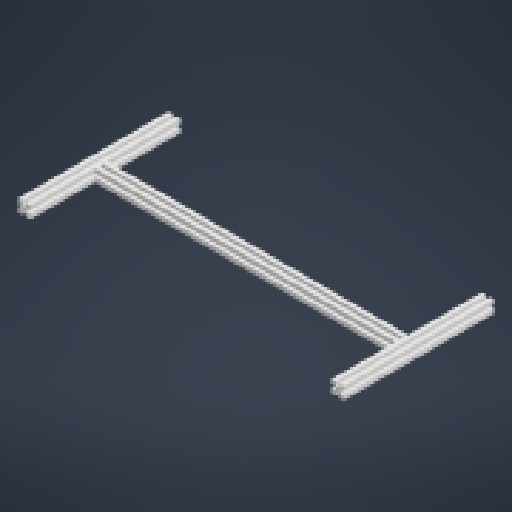
# Autodesk Inventor part: grabber
Saved by Autodesk Inventor 2024 (Build 280153000, 153)
## iProperties
Created: 2023-09-19
Part Number: grabber
Material: 일반
Document SubType Name: Modeling
Designer: 6gioc
Mass: 449.19 g
Surface Area: 2006.93 cm^2
Volume: 449.19 cm^3
Density: 1 g/cm^3
Appearance: 기본값
Author: 6gioc
Autodesk Inventor part; units mm, degrees
ref_plane "YZ Plane" through (0, 0, 0) normal (1, 0, 0) x (0, 1, 0)
ref_plane "XZ Plane" through (0, 0, 0) normal (0, 1, 0) x (-1, 0, 0)
ref_plane "XY Plane" through (0, 0, 0) normal (0, 0, 1) x (1, 0, 0)
sketch "스케치1" plane through (0, 0, 0) normal (0, 0, 1) x (1, 0, 0)
  line L0 (-15, 12.5) -> (5, 12.5)
  line L1 (5, 12.5) -> (5, -7.5)
  line L2 (5, -7.5) -> (-15, -7.5)
  line L3 (-15, -7.5) -> (-15, 12.5)
  line L4 (5, 5.25) -> (-0.5, 5.25)
  line L5 (-0.5, 5.25) -> (-0.5, -0.25)
  line L6 (-0.5, -0.25) -> (5, -0.25)
  line L7 (5, -0.25) -> (5, 5.25)
  line L8 (-7.75, 12.5) -> (-2.25, 12.5)
  line L9 (-2.25, 12.5) -> (-2.25, 7)
  line L10 (-2.25, 7) -> (-7.75, 7)
  line L11 (-7.75, 7) -> (-7.75, 12.5)
  line L12 (-15, 5.25) -> (-9.5, 5.25)
  line L13 (-9.5, 5.25) -> (-9.5, -0.25)
  line L14 (-9.5, -0.25) -> (-15, -0.25)
  line L15 (-15, -0.25) -> (-15, 5.25)
  line L16 (-7.75, -7.5) -> (-2.25, -7.5)
  line L17 (-2.25, -7.5) -> (-2.25, -2)
  line L18 (-2.25, -2) -> (-7.75, -2)
  line L19 (-7.75, -2) -> (-7.75, -7.5)
  line L20 (0, 0) -> (500, 0) projected
  line L21 (500, 0) -> (500, 5) projected
  line L22 (0, 5) -> (500, 5) projected
  line L23 (0, 0) -> (0, 5) projected
  line L24 (495, 12.5) -> (515, 12.5)
  line L25 (515, 12.5) -> (515, -7.5)
  line L26 (515, -7.5) -> (495, -7.5)
  line L27 (495, -7.5) -> (495, 12.5)
  line L28 (515, 5.25) -> (509.5, 5.25)
  line L29 (509.5, 5.25) -> (509.5, -0.25)
  line L30 (509.5, -0.25) -> (515, -0.25)
  line L31 (502.25, 12.5) -> (507.75, 12.5)
  line L32 (507.75, 12.5) -> (507.75, 7)
  line L33 (507.75, 7) -> (502.25, 7)
  line L34 (502.25, 7) -> (502.25, 12.5)
  line L35 (495, 5.25) -> (500.5, 5.25)
  line L36 (500.5, 5.25) -> (500.5, -0.25)
  line L37 (500.5, -0.25) -> (495, -0.25)
  line L38 (507.75, -7.5) -> (507.75, -2)
  line L39 (507.75, -2) -> (502.25, -2)
  line L40 (502.25, -2) -> (502.25, -7.5)
  dimension "d0" = 20
  dimension "d1" = 20
  dimension "d2" = 5.5
  dimension "d3" = 5.5
  dimension "d4" = 5.5
  dimension "d5" = 5.5
  dimension "d6" = 5.5
  dimension "d7" = 5.5
  dimension "d8" = 5.5
  dimension "d9" = 5.5
  dimension "d10" = 7.25
  dimension "d11" = 7.25
  dimension "d12" = 7.25
  dimension "d13" = 7.25
  dimension "d14" = 0.25
  dimension "d15" = 0.5
  dimension "d16" = 20
  dimension "d17" = 20
  dimension "d18" = 5.5
  dimension "d19" = 5.5
  dimension "d20" = 5.5
  dimension "d21" = 5.5
  dimension "d22" = 5.5
  dimension "d23" = 5.5
  dimension "d24" = 5.5
  dimension "d25" = 5.5
  dimension "d26" = 7.25
  dimension "d27" = 7.25
  dimension "d28" = 7.25
  dimension "d29" = 7.25
  dimension "d30" = 0.25
  dimension "d31" = 0.5
  constraints: 74 end point, 17 parallel, 9 horizontal, 9 perpendicular, 8 point on line
  measures "d0" distance of L1.end L2.end
  measures "d1" distance of L0.end L1.end
  measures "d2" distance of L6.end L5.end
  measures "d3" distance of L5.end L4.end
  measures "d4" distance of L9.end L10.end
  measures "d5" distance of L8.end L9.end
  measures "d6" distance of L13.end L14.end
  measures "d7" distance of L12.end L13.end
  measures "d8" distance of L18.end L17.end
  measures "d9" distance of L17.end L16.end
  measures "d10" distance between parallel lines of L1 L9
  measures "d11" distance between parallel lines of L0 L4
  measures "d12" distance between parallel lines of L1 L17
  measures "d13" distance between parallel lines of L0 L12
  measures "d14" distance between parallel lines of L4 L22
  measures "d15" distance between parallel lines of L23 L5
  measures "d16" distance of L25.end L27.start
  measures "d17" distance of L24.end L25.end
  measures "d18" distance of L30.end L29.end
  measures "d19" distance of L29.end L29.start
  measures "d20" distance of L32.end L34.start
  measures "d21" distance of L31.end L32.end
  measures "d22" distance of L36.end L37.end
  measures "d23" distance of L36.start L36.end
  measures "d24" distance of L40.start L39.start
  measures "d25" distance of L39.start L38.start
  measures "d26" distance between parallel lines of L25 L32
  measures "d27" distance between parallel lines of L24 L28
  measures "d28" distance between parallel lines of L25 L38
  measures "d29" distance between parallel lines of L24 L35
  measures "d30" distance between parallel lines of L37 L20
  measures "d31" distance between parallel lines of L36 L21
extrude "돌출1" add sketch "스케치1" against normal blind 140 contours L0 L11 L10 L9 L1 L4 L5 L6 L2 L17 L18 L19 L3 L14 L13 L12 | L27 L24 L34 L33 L32 L25 L28 L29 L30 L26 L38 L39 L40 L37 L36 L35
sketch "스케치2" plane through (0, 0, 0) normal (0, 0, 1) x (1, 0, 0)
  line L0 (-0.5, 5.25) -> (5, 5.25) projected
  line L1 (5, 5.25) -> (5, 12.5) projected
  line L2 (5, 12.5) -> (-2.25, 12.5) projected
  line L3 (-2.25, 12.5) -> (-2.25, 7) projected
  line L4 (-2.25, 7) -> (-7.75, 7) projected
  line L5 (-7.75, 7) -> (-7.75, 12.5) projected
  line L6 (-7.75, 12.5) -> (-15, 12.5) projected
  line L7 (-15, 12.5) -> (-15, 5.25) projected
  line L8 (-15, 5.25) -> (-9.5, 5.25) projected
  line L9 (-9.5, 5.25) -> (-9.5, -0.25) projected
  line L10 (-9.5, -0.25) -> (-15, -0.25) projected
  line L11 (-15, -0.25) -> (-15, -7.5) projected
  line L12 (-15, -7.5) -> (-7.75, -7.5) projected
  line L13 (-7.75, -7.5) -> (-7.75, -2) projected
  line L14 (-7.75, -2) -> (-2.25, -2) projected
  line L15 (-2.25, -2) -> (-2.25, -7.5) projected
  line L16 (-2.25, -7.5) -> (5, -7.5) projected
  line L17 (5, -7.5) -> (5, -0.25) projected
  line L18 (5, -0.25) -> (-0.5, -0.25) projected
  line L19 (-0.5, -0.25) -> (-0.5, 5.25) projected
  line L20 (502.25, 7) -> (502.25, 12.5) projected
  line L21 (502.25, 12.5) -> (495, 12.5) projected
  line L22 (495, 12.5) -> (495, 5.25) projected
  line L23 (495, 5.25) -> (500.5, 5.25) projected
  line L24 (500.5, 5.25) -> (500.5, -0.25) projected
  line L25 (500.5, -0.25) -> (495, -0.25) projected
  line L26 (495, -0.25) -> (495, -7.5) projected
  line L27 (495, -7.5) -> (502.25, -7.5) projected
  line L28 (502.25, -7.5) -> (502.25, -2) projected
  line L29 (502.25, -2) -> (507.75, -2) projected
  line L30 (507.75, -2) -> (507.75, -7.5) projected
  line L31 (507.75, -7.5) -> (515, -7.5) projected
  line L32 (515, -7.5) -> (515, -0.25) projected
  line L33 (515, -0.25) -> (509.5, -0.25) projected
  line L34 (509.5, -0.25) -> (509.5, 5.25) projected
  line L35 (509.5, 5.25) -> (515, 5.25) projected
  line L36 (515, 5.25) -> (515, 12.5) projected
  line L37 (515, 12.5) -> (507.75, 12.5) projected
  line L38 (507.75, 12.5) -> (507.75, 7) projected
  line L39 (507.75, 7) -> (502.25, 7) projected
  point P0 (0, 0)
extrude "돌출2" add sketch "스케치2" along normal blind 20
sketch "스케치3" plane through (495, 5.25, -140) normal (-1, 0, 0) x (0, 0, 1)
  line L0 (0, -12.75) -> (160, -12.75) projected
  line L1 (0, -5.5) -> (160, -5.5) projected
  line L2 (0, -12.75) -> (0, -5.5) projected
  line L3 (0, -12.75) -> (160, -12.75) projected
  line L4 (160, -5.5) -> (160, -12.75) projected
  line L5 (0, 7.25) -> (160, 7.25) projected
  line L6 (0, 0) -> (0, 7.25) projected
  line L7 (0, 0) -> (160, 0) projected
  line L8 (160, 7.25) -> (160, 0) projected
  line L9 (-360, -5.25) -> (140, -5.25) projected
  line L10 (140, -5.25) -> (140, -0.25) projected
  line L11 (-360, -0.25) -> (140, -0.25) projected
  line L12 (-360, -5.25) -> (-360, -0.25) projected
  line L13 (135, 7.25) -> (155, 7.25)
  line L14 (155, 7.25) -> (155, -12.75)
  line L15 (155, -12.75) -> (135, -12.75)
  line L16 (135, -12.75) -> (135, 7.25)
  line L17 (142.25, 7.25) -> (147.75, 7.25)
  line L18 (147.75, 7.25) -> (147.75, 1.75)
  line L19 (147.75, 1.75) -> (142.25, 1.75)
  line L20 (142.25, 1.75) -> (142.25, 7.25)
  line L21 (155, 0) -> (149.5, 0)
  line L22 (149.5, 0) -> (149.5, -5.5)
  line L23 (149.5, -5.5) -> (155, -5.5)
  line L24 (155, -5.5) -> (155, 0)
  line L25 (135, 0) -> (140.5, 0)
  line L26 (140.5, 0) -> (140.5, -5.5)
  line L27 (140.5, -5.5) -> (135, -5.5)
  line L28 (135, -5.5) -> (135, 0)
  line L29 (142.25, -12.75) -> (147.75, -12.75)
  line L30 (147.75, -12.75) -> (147.75, -7.25)
  line L31 (147.75, -7.25) -> (142.25, -7.25)
  line L32 (142.25, -7.25) -> (142.25, -12.75)
  line L33 (-360, -5.25) -> (140, -5.25) projected
  line L34 (140, -5.25) -> (140, -0.25) projected
  line L35 (-360, -0.25) -> (140, -0.25) projected
  line L36 (-360, -5.25) -> (-360, -0.25) projected
  line L37 (-360, -5.25) -> (140, -5.25) projected
  line L38 (140, -5.25) -> (140, -0.25) projected
  line L39 (-360, -0.25) -> (140, -0.25) projected
  line L40 (-360, -5.25) -> (-360, -0.25) projected
  line L41 (-360, -5.25) -> (140, -5.25) projected
  line L42 (140, -5.25) -> (140, -0.25) projected
  line L43 (-360, -0.25) -> (140, -0.25) projected
  line L44 (-360, -5.25) -> (-360, -0.25) projected
  point P0 (147.75, -12.75)
  point P1 (155, -5.5)
  point P2 (149.5, -5.5)
  point P3 (149.5, 0)
  point P4 (155, 0)
  point P5 (155, 7.25)
  point P6 (135, 0)
  point P7 (140.5, 0)
  point P8 (140.5, -5.5)
  point P9 (135, -12.75)
  dimension "d36" = 20
  dimension "d37" = 20
  dimension "d38" = 5.5
  dimension "d39" = 5.5
  dimension "d40" = 5.5
  dimension "d41" = 5.5
  dimension "d42" = 5.5
  dimension "d43" = 5.5
  dimension "d44" = 5.5
  dimension "d45" = 5.5
  dimension "d46" = 7.25
  dimension "d47" = 7.25
  dimension "d48" = 7.25
  dimension "d49" = 7.25
  dimension "d85" = 0.5
  constraints: 40 end point, 10 parallel, 5 horizontal, 5 perpendicular, 5 point on line
  measures "d36" distance of L14.end L15.end
  measures "d37" distance of L13.end L14.end
  measures "d38" distance of L18.end L19.end
  measures "d39" distance of L17.end L18.end
  measures "d40" distance of L23.end L22.end
  measures "d41" distance of L22.end L21.end
  measures "d42" distance of L26.end L27.end
  measures "d43" distance of L25.end L26.end
  measures "d44" distance of L31.end L30.end
  measures "d45" distance of L30.end L29.end
  measures "d46" distance between parallel lines of L16 L20
  measures "d47" distance between parallel lines of L13 L25
  measures "d48" distance between parallel lines of L13 L21
  measures "d49" distance between parallel lines of L14 L30
  measures "d85" distance between parallel lines of L26 L42
extrude "돌출3" add sketch "스케치3" along normal blind 490 contours L16 L1 L14 L0 L30 L31 L32 | L26 L7 L22 L1 | L7 L16 L5 L20 L19 L18 L14
sketch "스케치4" plane through (502.25, -7.5, -140) normal (0, -1, 0) x (1, 0, 0)
  line L0 (-517.25, 0) -> (-517.25, 160) projected
  line L1 (-510, 0) -> (-517.25, 0) projected
  line L2 (-510, 0) -> (-510, 160) projected
  line L3 (-517.25, 160) -> (-510, 160) projected
  line L4 (-497.25, 142.25) -> (-497.25, 147.75) projected
  line L5 (-7.25, 147.75) -> (-497.25, 147.75) projected
  line L6 (-7.25, 142.25) -> (-7.25, 147.75) projected
  line L7 (-7.25, 142.25) -> (-497.25, 142.25) projected
  line L8 (-7.25, 135) -> (-497.25, 135) projected
  line L9 (-7.25, 0) -> (-7.25, 135) projected
  line L10 (0, 0) -> (-7.25, 0) projected
  line L11 (0, 0) -> (0, 160) projected
  line L12 (-7.25, 160) -> (0, 160) projected
  line L13 (-7.25, 155) -> (-7.25, 160) projected
  line L14 (-7.25, 155) -> (-497.25, 155) projected
  line L15 (-497.25, 155) -> (-497.25, 160) projected
  line L16 (-504.5, 160) -> (-497.25, 160) projected
  line L17 (-504.5, 0) -> (-504.5, 160) projected
  line L18 (-497.25, 0) -> (-504.5, 0) projected
  line L19 (-497.25, 0) -> (-497.25, 135) projected
  line L20 (-510, 0) -> (-510, 160) projected
  line L21 (-504.5, 0) -> (-510, 0) projected
  line L22 (-504.5, 0) -> (-504.5, 160) projected
  line L23 (-510, 160) -> (-504.5, 160) projected
  line L24 (5.5, 0) -> (5.5, 160) projected
  line L25 (5.5, 0) -> (5.5, 160) projected
  line L26 (12.75, 0) -> (5.5, 0) projected
  line L27 (12.75, 0) -> (12.75, 160) projected
  line L28 (5.5, 160) -> (12.75, 160) projected
  line L29 (0, 0) -> (0, 160) projected
  line L30 (5.5, 0) -> (0, 0) projected
  line L31 (5.5, 0) -> (5.5, 160) projected
  line L32 (0, 160) -> (5.5, 160) projected
  line L33 (-517.25, 0) -> (-497.25, 0)
  line L34 (-497.25, 0) -> (-497.25, 20)
  line L35 (-497.25, 20) -> (-517.25, 20)
  line L36 (-517.25, 20) -> (-517.25, 0)
  line L37 (-517.25, 7.25) -> (-511.75, 7.25)
  line L38 (-511.75, 7.25) -> (-511.75, 12.75)
  line L39 (-511.75, 12.75) -> (-517.25, 12.75)
  line L40 (-517.25, 12.75) -> (-517.25, 7.25)
  line L41 (-510, 20) -> (-504.5, 20)
  line L42 (-504.5, 20) -> (-504.5, 14.5)
  line L43 (-504.5, 14.5) -> (-510, 14.5)
  line L44 (-510, 14.5) -> (-510, 20)
  line L45 (-510, 0) -> (-504.5, 0)
  line L46 (-504.5, 0) -> (-504.5, 5.5)
  line L47 (-504.5, 5.5) -> (-510, 5.5)
  line L48 (-510, 5.5) -> (-510, 0)
  line L49 (-497.25, 7.25) -> (-502.75, 7.25)
  line L50 (-502.75, 7.25) -> (-502.75, 12.75)
  line L51 (-502.75, 12.75) -> (-497.25, 12.75)
  line L52 (-497.25, 12.75) -> (-497.25, 7.25)
  line L53 (-7.25, 0) -> (12.75, 0)
  line L54 (12.75, 0) -> (12.75, 20)
  line L55 (12.75, 20) -> (-7.25, 20)
  line L56 (-7.25, 20) -> (-7.25, 0)
  line L57 (-7.25, 7.25) -> (-1.75, 7.25)
  line L58 (-1.75, 7.25) -> (-1.75, 12.75)
  line L59 (-1.75, 12.75) -> (-7.25, 12.75)
  line L60 (-7.25, 12.75) -> (-7.25, 7.25)
  line L61 (0, 20) -> (5.5, 20)
  line L62 (5.5, 20) -> (5.5, 14.5)
  line L63 (5.5, 14.5) -> (0, 14.5)
  line L64 (0, 14.5) -> (0, 20)
  line L65 (0, 0) -> (5.5, 0)
  line L66 (5.5, 0) -> (5.5, 5.5)
  line L67 (5.5, 5.5) -> (0, 5.5)
  line L68 (0, 5.5) -> (0, 0)
  line L69 (12.75, 7.25) -> (7.25, 7.25)
  line L70 (7.25, 7.25) -> (7.25, 12.75)
  line L71 (7.25, 12.75) -> (12.75, 12.75)
  line L72 (12.75, 12.75) -> (12.75, 7.25)
  point P0 (-502.25, 140)
  point P1 (-514.5, 12.75)
  point P2 (-510, 17.25)
  point P3 (-500, 12.75)
  point P4 (-4.5, 12.75)
  point P5 (0, 17.25)
  point P6 (10, 12.75)
  point P7 (12.75, 12.75)
  point P8 (5.5, 14.5)
  point P9 (0, 14.5)
  point P10 (0, 20)
  point P11 (-7.25, 12.75)
  point P12 (-7.25, 7.25)
  point P13 (0, 5.5)
  point P14 (5.5, 5.5)
  point P15 (12.75, 7.25)
  point P16 (-510, 5.5)
  point P17 (-504.5, 5.5)
  point P18 (-497.25, 7.25)
  point P19 (-497.25, 12.75)
  point P20 (-504.5, 14.5)
  point P21 (-510, 14.5)
  point P22 (-510, 20)
  point P23 (-517.25, 12.75)
  point P24 (-517.25, 7.25)
  dimension "d55" = 20
  dimension "d56" = 20
  dimension "d57" = 5.5
  dimension "d58" = 5.5
  dimension "d59" = 5.5
  dimension "d60" = 5.5
  dimension "d61" = 5.5
  dimension "d62" = 5.5
  dimension "d63" = 5.5
  dimension "d64" = 5.5
  dimension "d65" = 7.25
  dimension "d66" = 7.25
  dimension "d67" = 7.25
  dimension "d68" = 20
  dimension "d69" = 20
  dimension "d70" = 5.5
  dimension "d71" = 5.5
  dimension "d72" = 5.5
  dimension "d73" = 5.5
  dimension "d74" = 5.5
  dimension "d75" = 5.5
  dimension "d76" = 5.5
  dimension "d77" = 5.5
  dimension "d78" = 7.25
  dimension "d79" = 7.25
  constraints: 80 end point, 20 parallel, 11 horizontal, 10 perpendicular, 10 point on line, 6 midpoint
  measures "d55" distance of L35.end L34.end
  measures "d56" distance of L34.end L33.end
  measures "d57" distance of L39.end L38.end
  measures "d58" distance of L38.end L37.end
  measures "d59" distance of L42.end L43.end
  measures "d60" distance of L41.end L42.end
  measures "d61" distance of L47.end L46.end
  measures "d62" distance of L46.end L45.end
  measures "d63" distance of L50.end L51.end
  measures "d64" distance of L49.end L50.end
  measures "d65" distance from line of L35 point (-514.5, 12.75)
  measures "d66" distance from line of L0 point (-510, 17.25)
  measures "d67" distance from line of L35 point (-500, 12.75)
  measures "d68" distance of L56.start L55.start
  measures "d69" distance of L55.start L53.end
  measures "d70" distance of L59.end L58.end
  measures "d71" distance of L58.end L58.start
  measures "d72" distance of L63.start L63.end
  measures "d73" distance of L62.start L63.start
  measures "d74" distance of L68.start L67.start
  measures "d75" distance of L67.start L65.end
  measures "d76" distance of L70.end L71.end
  measures "d77" distance of L70.start L70.end
  measures "d78" distance from line of L55 point (-4.5, 12.75)
  measures "d79" distance from line of L55 point (10, 12.75)
extrude "돌출4" add sketch "스케치4" along normal blind 140 contours L0 L37 L38 L39 L35 L2 L1 | L2 L43 L17 L47 | L17 L35 L19 L51 L50 L49 L18 | L55 L11 L10 L9 L57 L58 L59 | L63 L24 L67 L11 | L55 L27 L71 L70 L69 L26 L24
sketch "스케치5" plane through (0, 0, -140) normal (0, 0, -1) x (-1, 0, 0)
  line L0 (-502.25, 12.5) -> (-495, 12.5) projected
  line L1 (-495, 12.5) -> (-495, 5.25) projected
  line L2 (-495, 5.25) -> (-500.5, 5.25) projected
  line L3 (-500.5, 5.25) -> (-500.5, -0.25) projected
  line L4 (-500.5, -0.25) -> (-495, -0.25) projected
  line L5 (-495, -0.25) -> (-495, -7.5) projected
  line L6 (-495, -7.5) -> (-502.25, -7.5) projected
  line L7 (-502.25, -7.5) -> (-502.25, -2) projected
  line L8 (-502.25, -2) -> (-507.75, -2) projected
  line L9 (-507.75, -2) -> (-507.75, -7.5) projected
  line L10 (-507.75, -7.5) -> (-515, -7.5) projected
  line L11 (-515, -7.5) -> (-515, -0.25) projected
  line L12 (-515, -0.25) -> (-509.5, -0.25) projected
  line L13 (-509.5, -0.25) -> (-509.5, 5.25) projected
  line L14 (-509.5, 5.25) -> (-515, 5.25) projected
  line L15 (-515, 5.25) -> (-515, 12.5) projected
  line L16 (-515, 12.5) -> (-507.75, 12.5) projected
  line L17 (-507.75, 12.5) -> (-507.75, 7) projected
  line L18 (-507.75, 7) -> (-502.25, 7) projected
  line L19 (-502.25, 7) -> (-502.25, 12.5) projected
  line L20 (-5, 5.25) -> (-5, 12.5) projected
  line L21 (-5, 12.5) -> (2.25, 12.5) projected
  line L22 (2.25, 12.5) -> (2.25, 7) projected
  line L23 (2.25, 7) -> (7.75, 7) projected
  line L24 (7.75, 7) -> (7.75, 12.5) projected
  line L25 (7.75, 12.5) -> (15, 12.5) projected
  line L26 (15, 12.5) -> (15, 5.25) projected
  line L27 (15, 5.25) -> (9.5, 5.25) projected
  line L28 (9.5, 5.25) -> (9.5, -0.25) projected
  line L29 (9.5, -0.25) -> (15, -0.25) projected
  line L30 (15, -0.25) -> (15, -7.5) projected
  line L31 (15, -7.5) -> (7.75, -7.5) projected
  line L32 (7.75, -7.5) -> (7.75, -2) projected
  line L33 (7.75, -2) -> (2.25, -2) projected
  line L34 (2.25, -2) -> (2.25, -7.5) projected
  line L35 (2.25, -7.5) -> (-5, -7.5) projected
  line L36 (-5, -7.5) -> (-5, -0.25) projected
  line L37 (-5, -0.25) -> (0.5, -0.25) projected
  line L38 (0.5, -0.25) -> (0.5, 5.25) projected
  line L39 (0.5, 5.25) -> (-5, 5.25) projected
  point P0 (0, 0)
extrude "돌출5" add sketch "스케치5" along normal blind 110
sketch "스케치6" plane through (5, 12.5, 15) normal (0, 1, 0) x (1, 0, 0)
  line L0 (490, 0) -> (0, 0) projected
  line L1 (235, 0) -> (255, 0)
  line L2 (255, 0) -> (255, 20)
  line L3 (255, 20) -> (235, 20)
  line L4 (235, 20) -> (235, 0)
  line L5 (0, 12.75) -> (0, 7.25) projected
  line L6 (490, 12.75) -> (0, 12.75) projected
  line L7 (490, 12.75) -> (490, 7.25) projected
  line L8 (490, 7.25) -> (0, 7.25) projected
  line L9 (490, 0) -> (0, 0) projected
  line L10 (490, 0) -> (490, -5) projected
  line L11 (497.25, -5) -> (490, -5) projected
  line L12 (497.25, 265) -> (497.25, -5) projected
  line L13 (490, 265) -> (497.25, 265) projected
  line L14 (490, 265) -> (490, 20) projected
  line L15 (490, 20) -> (0, 20) projected
  line L16 (0, 265) -> (0, 20) projected
  line L17 (-7.25, 265) -> (0, 265) projected
  line L18 (-7.25, 265) -> (-7.25, -5) projected
  line L19 (0, -5) -> (-7.25, -5) projected
  line L20 (0, 0) -> (0, -5) projected
  line L21 (235, 7.25) -> (240.5, 7.25)
  line L22 (240.5, 7.25) -> (240.5, 12.75)
  line L23 (240.5, 12.75) -> (235, 12.75)
  line L24 (235, 12.75) -> (235, 7.25)
  line L25 (255, 7.25) -> (249.5, 7.25)
  line L26 (249.5, 7.25) -> (249.5, 12.75)
  line L27 (249.5, 12.75) -> (255, 12.75)
  line L28 (255, 12.75) -> (255, 7.25)
  line L29 (242.25, 0) -> (247.75, 0)
  line L30 (247.75, 0) -> (247.75, 5.5)
  line L31 (247.75, 5.5) -> (242.25, 5.5)
  line L32 (242.25, 5.5) -> (242.25, 0)
  line L33 (242.25, 20) -> (247.75, 20)
  line L34 (247.75, 20) -> (247.75, 14.5)
  line L35 (247.75, 14.5) -> (242.25, 14.5)
  line L36 (242.25, 14.5) -> (242.25, 20)
  point P0 (-5, 15)
  point P1 (490, 10)
  point P2 (0, 10)
  point P3 (242.25, 17.25)
  point P4 (247.75, 0)
  point P5 (255, 0)
  point P6 (255, 7.25)
  point P7 (255, 12.75)
  point P8 (235, 12.75)
  point P9 (235, 7.25)
  dimension "d88" = 20
  dimension "d89" = 20
  dimension "d90" = 490
  dimension "d91" = 235
  dimension "d92" = 5.5
  dimension "d93" = 5.5
  dimension "d94" = 5.5
  dimension "d95" = 5.5
  dimension "d96" = 5.5
  dimension "d97" = 5.5
  dimension "d98" = 5.5
  dimension "d99" = 5.5
  dimension "d100" = 7.25
  dimension "d101" = 7.25
  dimension "d102" = 7.25
  dimension "d103" = 7.25
  constraints: 40 end point, 10 parallel, 5 horizontal, 5 perpendicular, 5 point on line, 3 midpoint
  measures "d88" distance of L3.end L2.end
  measures "d89" distance of L2.end L1.end
  measures "d90" distance of point (490, 10) point (0, 10)
  measures "d91" distance between parallel lines of L5 L4
  measures "d92" distance of L23.end L22.end
  measures "d93" distance of L22.end L21.end
  measures "d94" distance of L26.end L27.end
  measures "d95" distance of L25.end L26.end
  measures "d96" distance of L31.end L30.end
  measures "d97" distance of L30.end L29.end
  measures "d98" distance of L34.end L35.end
  measures "d99" distance of L33.end L34.end
  measures "d100" distance between parallel lines of L15 L23
  measures "d101" distance between parallel lines of L4 L32
  measures "d102" distance between parallel lines of L1 L25
  measures "d103" distance from line of L4 point (242.25, 17.25)
extrude "돌출6" add sketch "스케치6" along normal blind 300 contours L0 L30 L31 L32 L4 L8 L2 | L6 L4 L3 L36 L35 L34 L2 | L8 L22 L6 L26
